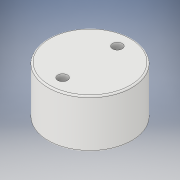
# Autodesk Inventor part: GU10-Socket
Saved by Autodesk Inventor 2018.2 (Build 222227000, 227)
## iProperties
Created: 2018-01-06
Part Number: GU10-Socket
Material: PC/ABS-Kunststoff
Document SubType Name: Modeling
Designer: JochenAlt
Density: 0.357273 g/cm^3
Appearance: Weiß
Author: JochenAlt
Autodesk Inventor part; units mm, degrees
ref_plane "YZ Plane" through (0, 0, 0) normal (1, 0, 0) x (0, 1, 0)
ref_plane "XZ Plane" through (0, 0, 0) normal (0, 1, 0) x (-1, 0, 0)
ref_plane "XY Plane" through (0, 0, 0) normal (0, 0, 1) x (1, 0, 0)
sketch "Skizze2" plane through (5, 0, 0) normal (0, 0, 1) x (0, 1, 0)
  line L0 (8.0381, 0) -> (-10.1665, 0) construction
  line L1 (0, 30.8) -> (0, -30.8) construction
  line L2 (-70, 0) -> (70, 0) construction
  arc A0 (3.0362, -5.7473) -> (1.6349, -3.0947) centre (2.3355, -4.421) ccw
  arc A1 (-3.0362, 5.7473) -> (-1.6349, 3.0947) centre (-2.3355, 4.421) ccw
  line L3 (-0.0061, 0) -> (9.6132, 0) construction
  line L4 (-0.0061, 0) -> (-9.6254, 0) construction
  circle A2 centre (0, 0) radius 5 construction
  line L5 (-2.3355, 4.421) -> (2.3355, -4.421) construction
  line L6 (-6.1863, -9.8413) -> (6.4207, 10.2142) construction
  arc A3 (-0.0105, -3.5) -> (-0.9975, -6.423) centre (-2.6609, -4.2331) ccw
  arc A4 (0.0105, 3.5) -> (0.9975, 6.423) centre (2.6609, 4.2331) ccw
  arc A5 (-10.5001, 0) -> (-10.5001, 0) centre (0, 0) ccw
  arc A6 (10.4999, 0) -> (10.4999, 0) centre (0, 0) ccw
  arc A7 (-7.5001, 0) -> (-7.5001, 0) centre (0, 0) ccw
  arc A8 (7.4999, 0) -> (7.4999, 0) centre (0, 0) ccw
  arc A9 (-0.0105, -3.5) -> (1.6349, -3.0947) centre (0, 0) ccw
  arc A10 (-0.9975, -6.423) -> (3.0362, -5.7473) centre (0, 0) ccw
  arc A11 (0.0105, 3.5) -> (-1.6349, 3.0947) centre (0, 0) ccw
  arc A12 (0.9975, 6.423) -> (-3.0362, 5.7473) centre (0, 0) ccw
  circle A13 centre (0, 0) radius 13.75
  circle A14 centre (0, 0) radius 12.75
  circle A15 centre (0, 0) radius 9 construction
  circle A16 centre (-9, 0) radius 1.6
  circle A17 centre (9, 0) radius 1.6
  arc A18 (-4.1245, -6.5613) -> (3.6201, -6.8526) centre (0, 0) ccw
  arc A19 (-3.5104, 6.9074) -> (-1.051, 1.9895) centre (-2.3355, 4.421) ccw
  arc A20 (3.6201, -6.8526) -> (1.051, -1.9895) centre (2.3355, -4.421) ccw
  arc A21 (-1.1974, -1.9049) -> (1.051, -1.9895) centre (0, 0) ccw
  arc A22 (1.1974, 1.9049) -> (-1.051, 1.9895) centre (0, 0) ccw
  arc A23 (4.1245, 6.5613) -> (-3.5104, 6.9074) centre (0.0019, 0.0031) ccw
  circle A24 centre (-9, 0) radius 2.75
  circle A25 centre (9, 0) radius 2.75
  dimension "d3" = 3
  dimension "d4" = 3
  dimension "d57" = 10
  dimension "d67" = 152.154
  dimension "d215" = 5.5
  dimension "d216" = 60
  dimension "d218" = 27.5
  dimension "d219" = 1
  dimension "d227" = 18
  dimension "d228" = 3.2
  dimension "d235" = 5.5
  constraints: 47 point on circle, 26 centre point, 22 point on line, 14 coincident, 10 end point, 5 tangent, 4 equal radius, 3 collinear, 2 midpoint, 1 horizontal, 1 other
  measures "d3" diameter of A0
  measures "d4" diameter of A1
  measures "d57" diameter of A2
  measures "d67" angle of L1 L5
  measures "d215" diameter of A3
  measures "d216" angle of L5 L6
  measures "d218" diameter of A13
  measures "d219" radial gap between concentric circles of A13 A14
  measures "d227" diameter of A15
  measures "d228" diameter of A16
  measures "d235" diameter of A24
extrude "Extrusion15" add sketch "Skizze2" along normal blind 16 contours A10 A3 A7 A9 A0 | A0 A9 A3 A21 A20 A7 A10 | A7 A20 A18 A3 | A3 A7 | A3 A7 A24 A19 A22 A4 A25 A20 A21 | A18 A20 A7 A25 A5 A24 A3 | A24 A5 A16 A7 | A7 A16 A24 | A25 A7 A17 | A7 A17 A5 A25 | A24 A5 A16 | A25 A5 A17 A7 | A7 A4 A23 A19 A24 A5 A25 | A5 A17 A25 | A16 A5 A24 A7 | A7 A4 | A4 A11 A1 A12 A7 | A19 A23 A4 A7 | A7 A4 A12 A1 A11 A22 A19 | A13 | A14
extrude "Extrusion16" cut sketch "Skizze2" along normal blind 5.5 contours A10 A3 A7 A9 A0 | A0 A9 A3 A21 A20 A7 A10 | A7 A20 A18 A3 | A3 A7 | A3 A7 A24 A19 A22 A4 A25 A20 A21 | A18 A20 A7 A25 A5 A24 A3 | A24 A5 A16 A7 | A7 A16 A24 | A25 A7 A17 | A7 A17 A5 A25 | A16 A5 A7 | A7 A16 | A24 A5 A16 | A17 A7 | A7 A17 A5 | A25 A5 A17 A7 | A7 A4 A23 A19 A24 A5 A25 | A5 A17 A25 | A16 A5 A24 A7 | A16 A5 | A5 A17 | A7 A4 | A4 A11 A1 A12 A7 | A19 A23 A4 A7 | A7 A4 A12 A1 A11 A22 A19 | A14
extrude "Extrusion17" cut sketch "Skizze2" along normal blind 9 contours A10 A3 A7 A9 A0 | A3 A7 | A7 A4 | A4 A11 A1 A12 A7
extrude "Extrusion19" cut sketch "Skizze2" against normal blind 4 from surface at 9 contours A0 A9 A3 A21 A20 A7 A10 | A7 A20 A18 A3 | A19 A23 A4 A7 | A7 A4 A12 A1 A11 A22 A19
extrude "Extrusion20" cut sketch "Skizze2" along normal blind 3 from surface at 5.5 contours A24 A5 A16 A7 | A7 A16 A24 | A25 A7 A17 | A7 A17 A5 A25 | A24 A5 A16 | A25 A5 A17 A7 | A5 A17 A25 | A16 A5 A24 A7
fillet "Rundung8" radius 1 1 edges at (5, -12.75, 5.5)
fillet "Rundung9" radius 0.5 3 edges at (5, -13.75, 16) (5, -13.75, 0) (5, -12.75, 0)
equation "\"d4\" = d3"
equation "\"d91\" = 60deg"
equation "\"Skizze5_Pitch\" = 2"
equation "\"d111\" = 60deg"
equation "\"Skizze7_Pitch\" = 2"
equation "\"d129\" = 60deg"
equation "\"Skizze9_Pitch\" = 2"
equation "\"d147\" = 60deg"
equation "\"Skizze11_Pitch\" = 2.5"
equation "\"d165\" = 60deg"
equation "\"Skizze13_Pitch\" = 2"
